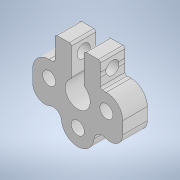
# Autodesk Inventor part: カップリング_軸6mm
Saved by Autodesk Inventor 2021 (Build 250183000, 183)
## iProperties
Created: 2022-01-31
Part Number: カップリング_軸6mm
Material: 一般
Document SubType Name: Modeling
Designer: hirohumi
Density: 1 g/cm^3
Appearance: 既定
Author: hirohumi
Autodesk Inventor part; units mm, degrees
ref_plane "YZ Plane" through (0, 0, 0) normal (1, 0, 0) x (0, 1, 0)
ref_plane "XZ Plane" through (0, 0, 0) normal (0, 1, 0) x (-1, 0, 0)
ref_plane "XY Plane" through (0, 0, 0) normal (0, 0, 1) x (1, 0, 0)
sketch "スケッチ1" plane through (0, 0, 0) normal (0, 0, 1) x (1, 0, 0)
  arc A0 (-1.55, 2.6268) -> (1.55, 2.6268) centre (0, 0) ccw
  circle A1 centre (-7, 0) radius 1.6
  circle A2 centre (7, 0) radius 1.6
  arc A3 (-7, 4) -> (-11, 0) centre (-7, 0) ccw
  arc A4 (11, 0) -> (7, 4) centre (7, 0) ccw
  line L0 (-1.55, 10) -> (-1.55, 2.6268)
  line L1 (1.55, 10) -> (1.55, 2.6268)
  circle A5 centre (0, -7) radius 1.6
  line L2 (1.55, 10) -> (5.55, 10)
  line L3 (5.55, 10) -> (5.55, 7.5385)
  line L4 (5.55, 4) -> (7, 4)
  line L5 (-1.55, 10) -> (-5.55, 10)
  line L6 (-5.55, 10) -> (-5.55, 7.5385)
  line L7 (-5.55, 4) -> (-7, 4)
  line L8 (-11, 0) -> (-11, -3)
  arc A6 (-11, -3) -> (-6.7837, -5.7424) centre (-8, -3) ccw
  arc A7 (1.55, 2.6268) -> (-1.55, 2.6268) centre (0, 0) ccw construction
  arc A8 (-3.9819, -7.3804) -> (3.9819, -7.3804) centre (0, -7) ccw
  arc A9 (-3.9819, -7.3804) -> (-6.7837, -5.7424) centre (-5.9728, -7.5706) ccw
  line L9 (11, 0) -> (11, -3)
  arc A10 (6.7837, -5.7424) -> (11, -3) centre (8, -3) ccw
  arc A11 (6.7837, -5.7424) -> (3.9819, -7.3804) centre (5.9728, -7.5706) ccw
  arc A12 (-5.55, 7.5385) -> (-5.55, 6.4615) centre (-6.95, 7) ccw construction
  arc A13 (5.55, 6.4615) -> (5.55, 7.5385) centre (6.95, 7) ccw construction
  arc A14 (-5.55, 6.4615) -> (-5.55, 7.5385) centre (-6.95, 7) ccw
  arc A15 (5.55, 7.5385) -> (5.55, 6.4615) centre (6.95, 7) ccw
  line L10 (5.55, 6.4615) -> (5.55, 4)
  line L11 (5.55, 7.5385) -> (5.55, 6.4615) construction
  line L12 (-5.55, 6.4615) -> (-5.55, 4)
  line L13 (-5.55, 7.5385) -> (-5.55, 6.4615) construction
  dimension "d0" = 6.1
  dimension "d1" = 3.2
  dimension "d2" = 3.2
  dimension "d4" = 7
  dimension "d5" = 7
  dimension "d6" = 3.2
  dimension "d7" = 7
  dimension "d8" = 6
  dimension "d9" = 4
  dimension "d10" = 3.1
  dimension "d11" = 4
  dimension "d12" = 4
  dimension "d13" = 1.55
  dimension "d14" = 3
  dimension "d15" = 3
  dimension "d16" = 4
  dimension "d17" = 4
  dimension "d18" = 3
  dimension "d19" = 3
  dimension "d20" = 2
  dimension "d21" = 2
  dimension "d22" = 3
  dimension "d23" = 3
  dimension "d24" = 1.4
  dimension "d25" = 1.4
  dimension "d26" = 3
  dimension "d27" = 3
  constraints: 28 end point, 26 point on circle, 16 centre point, 10 tangent, 6 perpendicular, 4 coincident, 4 vertical, 3 horizontal, 2 horizontal alignment, 1 point on line, 1 vertical alignment
  measures "d0" diameter of A0
  measures "d1" diameter of A1
  measures "d2" diameter of A2
  measures "d4" distance of point (0, 0) A1.centre
  measures "d5" distance of A2.centre point (0, 0)
  measures "d6" diameter of A5
  measures "d7" distance of A5.centre point (0, 0)
  measures "d8" distance between parallel lines of L7 L5
  measures "d9" radius of A3
  measures "d10" distance between parallel lines of L1 L0
  measures "d11" distance of L0.start L5.end
  measures "d12" distance of L1.start L2.end
  measures "d13" distance from line of point (0, 0) L0
  measures "d14" distance of L8.start L8.end
  measures "d15" radius of A6
  measures "d16" radius of A8
  measures "d17" radius of A4
  measures "d18" distance of L9.start L9.end
  measures "d19" radius of A10
  measures "d20" radius of A11
  measures "d21" radius of A9
  measures "d22" diameter of A12
  measures "d23" diameter of A13
  measures "d24" distance from line of A13.centre L3
  measures "d25" distance from line of L6 A12.centre
  measures "d26" distance from line of L2 A13.centre
  measures "d27" distance from line of L5 A12.centre
extrude "押し出し1" add sketch "スケッチ1" along normal blind 6
sketch "スケッチ2" plane through (5.55, 4, 0) normal (1, 0, 0) x (0, 0, -1)
  circle A0 centre (-3, 3) radius 1.6
  line L0 (0, 6) -> (-6, 6) projected
  point P0 (0, -4)
  dimension "d30" = 3.2
  dimension "d31" = 3
  dimension "d32" = 3
  constraints: 1 centre point
  measures "d30" diameter of A0
  measures "d31" distance from line of L0 A0.centre
  measures "d32" horizontal distance of L0.start A0.centre
extrude "押し出し2" cut sketch "スケッチ2" against normal through all
fillet "フィレット1" radius 0.5 8 edges at (-5.55, 10, 3) (-1.55, 10, 3) (1.55, 10, 3) (5.55, 10, 3) (5.55, 4, 3) (-5.55, 4, 3) (-1.55, 2.6268, 3) (1.55, 2.6268, 3)
